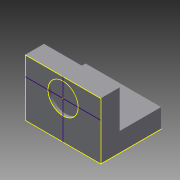
# Autodesk Inventor part: camera
Saved by Autodesk Inventor 2014 (Build 180170000, 170)
## iProperties
Created: 2014-03-23
Part Number: camera
Material: Generic
Document SubType Name: Modeling
Designer: jferner
Density: 1 g/cm^3
Appearance: Default
cameraLensHeight: 1.250 in
cameraMountingHoleDistanceFromFront: 1.125 in
cameraWidth: 2.500 in
cameraDepth: 2.000 in
cameraMountingHoleDepth: 0.332 in
Author: jferner
Autodesk Inventor part; units mm, degrees
ref_plane "YZ Plane" through (0, 0, 0) normal (1, 0, 0) x (0, 1, 0)
ref_plane "XZ Plane" through (0, 0, 0) normal (0, 1, 0) x (-1, 0, 0)
ref_plane "XY Plane" through (0, 0, 0) normal (0, 0, 1) x (1, 0, 0)
sketch "Sketch1" plane through (0, 0, 0) normal (0, 1, 0) x (-1, 0, 0)
  line L0 (0, 0) -> (63.5, 0)
  line L1 (63.5, 0) -> (63.5, 50.8)
  line L2 (63.5, 50.8) -> (0, 50.8)
  line L3 (0, 50.8) -> (0, 0)
  dimension "cameraWidth" = 63.5
  dimension "cameraDepth" = 50.8
  constraints: 8 end point, 2 parallel, 1 horizontal, 1 perpendicular
  measures "cameraWidth" distance of L1.end L2.end
  measures "cameraDepth" distance of L0.end L1.end
extrude "Extrusion1" add sketch "Sketch1" along normal blind 15.875
sketch "Sketch2" plane through (0, 15.875, 0) normal (0, 1, 0) x (1, 0, 0)
  line L0 (0, -50.8) -> (0, 0) projected
  line L1 (-63.5, -50.8) -> (0, -50.8)
  line L2 (0, -50.8) -> (0, -34.925)
  line L3 (0, -34.925) -> (-63.5, -34.925)
  line L4 (-63.5, -34.925) -> (-63.5, -50.8)
  dimension "d4" = 15.875
  constraints: 8 end point, 2 parallel, 1 horizontal, 1 perpendicular, 1 point on line
  measures "d4" distance between parallel lines of L1 L3
extrude "Extrusion2" add sketch "Sketch2" along normal blind 31.75
sketch "Sketch3" plane through (-63.5, 0, 50.8) normal (0, 0, 1) x (1, 0, 0)
  line L0 (0, 0) -> (63.5, 0) projected
  line L1 (0, 0) -> (0, 47.625) projected
  circle A0 centre (31.75, 31.75) radius 12.7
  dimension "d7" = 31.75
  dimension "cameraLensHeight" = 31.75
  dimension "d9" = 25.4
  constraints: 1 centre point
  measures "d7" distance from line of L1 A0.centre
  measures "cameraLensHeight" distance from line of L0 A0.centre
  measures "d9" diameter of A0
extrude "Extrusion3" cut sketch "Sketch3" against normal blind 2.54
sketch "Sketch4" plane through (-63.5, 0, 50.8) normal (0, 0, 1) x (1, 0, 0)
  circle A0 centre (31.75, 31.75) radius 12.7 projected
  line L0 (0, 0) -> (63.5, 0) projected
  line L1 (63.5, 0) -> (63.5, 47.625) projected
  line L2 (0, 47.625) -> (63.5, 47.625) projected
  line L3 (0, 0) -> (0, 47.625) projected
  line L4 (0, 31.75) -> (63.5, 31.75)
  line L5 (31.75, 47.625) -> (31.75, 0)
  dimension "d12" = 31.75
  constraints: 4 end point, 2 midpoint, 2 point on line, 1 perpendicular
  measures "d12" distance between parallel lines of L0 L4
sketch "Sketch5" plane through (0, 0, 0) normal (0, -1, 0) x (1, 0, 0)
  line L0 (0, 0) -> (-63.5, 0) projected
  line L1 (0, 50.8) -> (0, 0) projected
  line L2 (-63.5, 50.8) -> (0, 50.8) projected
  line L3 (-63.5, 0) -> (-63.5, 50.8) projected
  line L4 (-63.5, 22.225) -> (0, 22.225)
  line L5 (-31.75, 50.8) -> (-31.75, 0)
  circle A0 centre (-31.75, 22.225) radius 7.8401
  dimension "cameraMountingHoleDistanceFromFront" = 28.575
  constraints: 4 end point, 3 midpoint, 3 point on line, 1 centre point, 1 perpendicular
  measures "cameraMountingHoleDistanceFromFront" distance between parallel lines of L2 L4
hole "Hole1" at (-31.75, 0, 22.225) direction (0, 1, 0) diameter 4.9784 depth 8.43 thread size "1/4-20 UNC" class "2B" standard "ANSI Unified Screw Threads"
equation "\"d7\" = 0.5 * cameraWidth"
equation "\"d12\" = cameraLensHeight"
body "Solid1"
